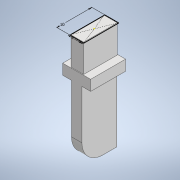
# Autodesk Inventor part: lavalier_holder
Saved by Autodesk Inventor 2022 (Build 260153070, 153G)
## iProperties
Created: 2021-06-08
Part Number: lavalier_holder
Material: Generic
Document SubType Name: Modeling
Designer: fraaw
Density: 1 g/cm^3
Appearance: Default
Author: fraaw
Autodesk Inventor part; units mm, degrees
ref_plane "YZ Plane" through (0, 0, 0) normal (1, 0, 0) x (0, 1, 0)
ref_plane "XZ Plane" through (0, 0, 0) normal (0, 1, 0) x (-1, 0, 0)
ref_plane "XY Plane" through (0, 0, 0) normal (0, 0, 1) x (1, 0, 0)
sketch "Sketch1" plane through (0, 0, 0) normal (0, 1, 0) x (-1, 0, 0)
  line L0 (-1.8, -4.8) -> (1.8, -4.8)
  line L1 (1.8, -4.8) -> (1.8, 4.8)
  line L2 (1.8, 4.8) -> (-1.8, 4.8)
  line L3 (-1.8, 4.8) -> (-1.8, -4.8)
  line L4 (-1.8, -4.8) -> (1.8, 4.8) construction
  line L5 (1.8, -4.8) -> (-1.8, 4.8) construction
  point P0 (0, 0)
  dimension "d0" = 3.6
  dimension "d1" = 9.6
  constraints: 12 end point, 2 midpoint, 2 parallel, 1 horizontal, 1 perpendicular
  measures "d0" distance of L1.end L2.end
  measures "d1" distance of L2.end L0.start
extrude "Extrusion1" add sketch "Sketch1" along normal blind 8
sketch "Sketch2" plane through (0, 0, 0) normal (0, -1, 0) x (1, 0, 0)
  line L0 (-4, -5) -> (4, -5)
  line L1 (4, -5) -> (4, 5)
  line L2 (4, 5) -> (-4, 5)
  line L3 (-4, 5) -> (-4, -5)
  line L4 (-4, -5) -> (4, 5) construction
  line L5 (4, -5) -> (-4, 5) construction
  point P0 (0, 0)
  dimension "d4" = 8
  dimension "d5" = 10
  constraints: 12 end point, 2 midpoint, 2 parallel, 1 horizontal, 1 perpendicular
  measures "d4" distance of L1.end L2.end
  measures "d5" distance of L0.end L1.end
extrude "Extrusion2" add sketch "Sketch2" along normal blind 23
fillet "Fillet1" radius 6 1 edges at (0, -23, 5)
sketch "Sketch3" plane through (4, 0, -5) normal (0, 0, -1) x (-1, 0, 0)
  line L0 (0, 0) -> (0, -17) projected
  line L1 (8, -23) -> (0, -23) projected
  line L2 (0, -3) -> (0, -23)
  line L3 (0, -23) -> (2.5, -23)
  line L4 (2.5, -23) -> (2.5, -3)
  line L5 (2.5, -3) -> (0, -3)
  line L6 (8, 0) -> (0, 0) projected
  line L7 (4, 0) -> (4, -23) construction
  line L8 (8, -3) -> (8, -23)
  line L9 (8, -23) -> (5.5, -23)
  line L10 (5.5, -23) -> (5.5, -3)
  line L11 (5.5, -3) -> (8, -3)
  point P0 (8, -17)
  dimension "d9" = 1.5
  dimension "d10" = 3
  constraints: 18 end point, 4 symmetric about line, 2 parallel, 2 perpendicular, 1 midpoint, 1 point on line
  measures "d9" distance from line of L4 L7.start
  measures "d10" distance between parallel lines of L5 L6
extrude "Extrusion3" cut sketch "Sketch3" against normal up to next
sketch "Sketch4" plane through (0, 8, 0) normal (0, 1, 0) x (1, 0, 0)
  line L0 (2, 5) -> (-2, 5)
  line L1 (-2, 5) -> (-2, -5)
  line L2 (-2, -5) -> (2, -5)
  line L3 (2, -5) -> (2, 5)
  line L4 (2, 5) -> (-2, -5) construction
  line L5 (-2, 5) -> (2, -5) construction
  point P0 (0, 0)
  dimension "d13" = 4
  dimension "d14" = 10
  constraints: 12 end point, 2 midpoint, 2 parallel, 1 horizontal, 1 perpendicular
  measures "d13" distance of L1.end L2.end
  measures "d14" distance of L0.end L1.end
body "Solid1"
